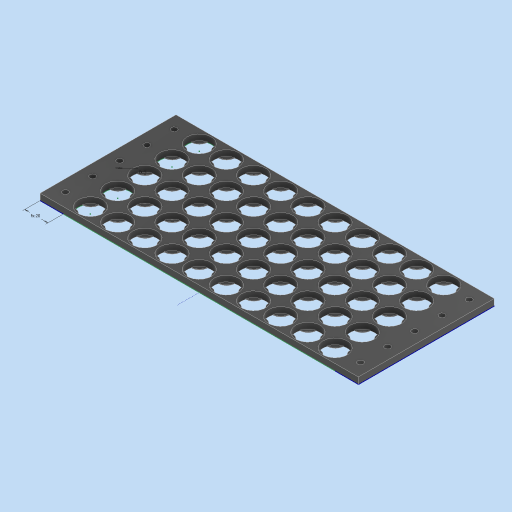
# Autodesk Inventor part: CO-2-1_CellSpacerBottom
Saved by Autodesk Inventor 2023 (Build 270158000, 158)
## iProperties
Created: 2022-10-25
Part Number: CO-2-1_CellSpacerBottom
Material: Generic
Document SubType Name: Modeling
Designer: asach
Density: 1 g/cm^3
Appearance: Dark Gray
Author: asach
Autodesk Inventor part; units mm, degrees
ref_plane "YZ Plane" through (0, 0, 0) normal (1, 0, 0) x (0, 1, 0)
ref_plane "XZ Plane" through (0, 0, 0) normal (0, 1, 0) x (-1, 0, 0)
ref_plane "XY Plane" through (0, 0, 0) normal (0, 0, 1) x (1, 0, 0)
sketch "Sketch1" plane through (0, 0, 0) normal (0, 1, 0) x (-1, 0, 0)
  circle A0 centre (0, 0) radius 10.5
  line L0 (-11.7, 11.7) -> (11.7, 11.7)
  line L1 (11.7, 11.7) -> (11.7, -11.7)
  line L2 (11.7, -11.7) -> (-11.7, -11.7)
  line L3 (-11.7, -11.7) -> (-11.7, 11.7)
  line L4 (-11.7, 11.7) -> (11.7, -11.7) construction
  line L5 (11.7, 11.7) -> (-11.7, -11.7) construction
  line L6 (-10.4975, -0.2304) -> (0.2823, 10.4962)
  line L7 (-11.7, 3.294) -> (-3.0039, 11.7)
  arc A1 (-11.7, 3.294) -> (-3.0039, 11.7) centre (-10.1198, 10.3604) ccw
  arc A2 (-3.294, -11.7) -> (-11.7, -3.0039) centre (-10.3604, -10.1198) ccw
  line L8 (-3.294, -11.7) -> (-11.7, -3.0039)
  arc A3 (11.7, -3.294) -> (3.0039, -11.7) centre (10.1198, -10.3604) ccw
  line L9 (11.7, -3.294) -> (3.0039, -11.7)
  arc A4 (3.294, 11.7) -> (11.7, 3.0039) centre (10.3604, 10.1198) ccw
  line L10 (3.294, 11.7) -> (11.7, 3.0039)
  point P0 (-2.8837, 10.0963)
  point P1 (3.1201, 10.0257)
  point P2 (10.0963, 2.8837)
  point P3 (10.0257, -3.1201)
  point P4 (2.8837, -10.0963)
  point P5 (-3.1201, -10.0257)
  point P6 (-10.0963, -2.8837)
  point P7 (-10.0257, 3.1201)
  dimension "d0" = 21
  dimension "d1" = 23.4
  dimension "d6" = 360
  constraints: 22 end point, 10 point on circle, 5 centre point, 2 midpoint, 2 parallel, 2 perpendicular, 2 point on line, 2 tangent, 1 coincident, 1 horizontal, 21 other
  measures "d0" diameter of A0
  measures "d1" distance of L0.end L1.end
extrude "Extrusion1" add sketch "Sketch1" along normal blind 5 contours A0 A4 L1 A3 | A0 L10 A4 | A3 L9 A0 | A0 A4 L10 | L10 L0 L1 | A0 A1 L0 A4 | L9 A3 A0 | L9 L1 L2 | A3 L2 A2 A0 | A2 L8 A0 | L7 L3 L0 | A1 A0 L7 | L2 L3 L8 | L8 A2 A0 | A2 L3 A1 A0 | A0 A1 L7
extrude "Extrusion2" add sketch "Sketch1" against normal blind 0.5 contours A0 A4 L1 A3 | A4 A0 | A0 L10 A4 | A3 L9 A0 | A0 A3 | A0 A4 L10 | L10 L0 L1 | A0 A1 L0 A4 | L9 A3 A0 | L9 L1 L2 | A3 L2 A2 A0 | A2 L8 A0 | A0 A2 | L7 L3 L0 | A1 A0 L7 | A1 A0 | L2 L3 L8 | L8 A2 A0 | A2 L3 A1 A0 | A0 A1 L7
pattern_linear "Rectangular Pattern1" count 10 spacing 23.4 along (1, 0, 0) count 5 spacing 23.4 along (0, 0, 1)
sketch "Sketch2" plane through (0, -0.5, 0) normal (0, -1, 0) x (1, 0, 0)
  line L0 (-11.7, 105.3) -> (-11.7, -11.7) projected
  line L1 (222.3, -11.7) -> (222.3, 105.3) projected
  line L2 (-11.7, -11.7) -> (-11.7, 105.3) projected
  line L3 (-11.7, 105.3) -> (-31.7, 105.3)
  line L4 (-31.7, 105.3) -> (-31.7, -11.7)
  line L5 (-31.7, -11.7) -> (-11.7, -11.7)
  line L6 (-11.7, -11.7) -> (-11.7, 105.3)
  line L7 (-11.7, 105.3) -> (222.3, 105.3) projected
  line L8 (222.3, 105.3) -> (242.3, 105.3)
  line L9 (242.3, 105.3) -> (242.3, -11.7)
  line L10 (242.3, -11.7) -> (222.3, -11.7)
  line L11 (222.3, -11.7) -> (222.3, 105.3)
  line L12 (-21.7, 105.3) -> (-21.7, -11.7) construction
  line L13 (-31.7, 46.8) -> (-11.7, 46.8) construction
  circle A0 centre (-21.7, 46.8) radius 2.5
  arc A1 (-10.0963, 73.0837) -> (-10.0257, 67.0799) centre (0, 70.2) ccw projected
  arc A2 (-10.0963, 96.4837) -> (-10.0257, 90.4799) centre (0, 93.6) ccw projected
  arc A3 (-10.0963, 26.2837) -> (-10.0257, 20.2799) centre (0, 23.4) ccw projected
  arc A4 (-10.0963, 2.8837) -> (-10.0257, -3.1201) centre (0, 0) ccw projected
  circle A5 centre (0, 0) radius 10.5 projected
  line L14 (-10.4993, -0.1233) -> (-31.7, -0.1233) construction
  line L15 (-10.4993, 23.2767) -> (-31.7, 23.2767) construction
  circle A6 centre (0, 70.2) radius 10.5 projected
  line L16 (-10.4993, 70.0767) -> (-31.7, 70.0767) construction
  line L17 (-10.4993, 93.4767) -> (-31.7, 93.4767) construction
  circle A7 centre (-21.7, 93.4767) radius 2.5
  circle A8 centre (-21.7, 70.0767) radius 2.5
  circle A9 centre (-21.7, 23.2767) radius 2.5
  circle A10 centre (-21.7, -0.1233) radius 2.5
  line L18 (222.3, 105.3) -> (-11.7, 105.3) projected
  line L19 (105.3, 105.3) -> (105.3, 124.5019) construction
  circle A11 centre (232.3, 46.8) radius 2.5
  circle A12 centre (232.3, 93.4767) radius 2.5
  circle A13 centre (232.3, 70.0767) radius 2.5
  circle A14 centre (232.3, 23.2767) radius 2.5
  circle A15 centre (232.3, -0.1233) radius 2.5
  dimension "d16" = 20
  dimension "d17" = 5
  constraints: 30 end point, 13 point on line, 10 centre point, 6 midpoint, 6 perpendicular, 6 point on circle, 5 symmetric about line, 4 equal radius, 4 parallel, 2 horizontal, 1 collinear, 1 vertical, 5 other
  measures "d16" distance of L0.start L3.end
  measures "d17" diameter of A0
extrude "Extrusion3" add sketch "Sketch2" against normal up to surface (5.5 mm away) contours L0 L5 L4 L3 | L8 L9 L10 L1
equation "\"d16\" = screwTabWidth"
equation "\"d17\" = screwDiameter"
equation "\"cellSpacing\" = 1.2"
equation "\"screwTabWidth\" = 20"
equation "\"screwDiameter\" = 5"
body "Solid1"
